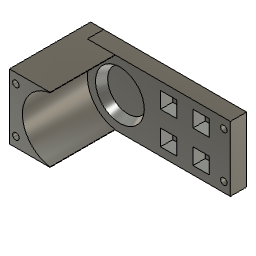
cementform_circle_80x40_plateA (Autodesk Fusion 360 design; units mm, degrees)
Autodesk Fusion 360 part; units mm, degrees
sketch "baseplate" plane through (0, 0, 0) normal (0, 1, 0) x (1, 0, 0)
  line L0 (0, 0) -> (80, 0)
  line L1 (80, 0) -> (80, -40)
  line L2 (80, -40) -> (0, -40)
  line L3 (0, -40) -> (0, 0)
  dimension "d1" = 40
  dimension "d2" = 80
  constraint horizontal L0
  constraint vertical L1
  constraint horizontal L2
  constraint vertical L3
  constraint coincident L0.start L3.end
  measures "d1" distance of L0.start L2.end
  measures "d2" distance of L0.start L0.end
extrude "Extrude1" add sketch "baseplate" along normal blind 10
sketch "outside_pryamid" plane through (0, 0, 0) normal (0, 1, 0) x (1, 0, 0)
  line L0 (45, -35) -> (55, -35)
  line L1 (55, -35) -> (55, -25)
  line L2 (55, -25) -> (45, -25)
  line L3 (45, -25) -> (45, -35)
  line L4 (65, -35) -> (75, -35)
  line L5 (75, -35) -> (75, -25)
  line L6 (75, -25) -> (65, -25)
  line L7 (65, -25) -> (65, -35)
  line L8 (45, -15) -> (55, -15)
  line L9 (55, -15) -> (55, -5)
  line L10 (55, -5) -> (45, -5)
  line L11 (45, -5) -> (45, -15)
  line L12 (65, -15) -> (75, -15)
  line L13 (75, -15) -> (75, -5)
  line L14 (75, -5) -> (65, -5)
  line L15 (65, -5) -> (65, -15)
  circle A0 centre (20, -20) radius 15
  dimension "d40" = 30
  constraint horizontal L0
  constraint vertical L1
  constraint horizontal L2
  constraint vertical L3
  constraint horizontal L4
  constraint vertical L5
  constraint horizontal L6
  constraint vertical L7
  constraint horizontal L8
  constraint vertical L9
  constraint horizontal L10
  constraint vertical L11
  constraint horizontal L12
  constraint vertical L13
  constraint horizontal L14
  constraint vertical L15
  measures "d40" diameter of A0
ref_plane "WorkPlane1" through (0, 5, 0) normal (0, 1, 0) x (0, 0, 1)
sketch "inside_pryamid" plane through (0, 5, 0) normal (0, 1, 0) x (1, 0, 0)
  line L0 (47.5, -7.5) -> (47.5, -10)
  line L1 (47.5, -12.5) -> (52.5, -12.5)
  line L2 (52.5, -7.5) -> (47.5, -7.5)
  line L3 (47.5, -10) -> (47.5, -12.5)
  line L4 (52.5, -12.5) -> (52.5, -7.5)
  line L5 (67.5, -10) -> (67.5, -12.5)
  line L6 (67.5, -12.5) -> (72.5, -12.5)
  line L7 (67.5, -7.5) -> (67.5, -10)
  line L8 (72.5, -12.5) -> (72.5, -7.5)
  line L9 (72.5, -7.5) -> (67.5, -7.5)
  line L10 (67.5, -10) -> (67.5, -12.5)
  line L11 (67.5, -12.5) -> (72.5, -12.5)
  line L12 (72.5, -12.5) -> (72.5, -7.5)
  line L13 (47.5, -7.5) -> (47.5, -10)
  line L14 (52.5, -12.5) -> (52.5, -7.5)
  line L15 (72.5, -7.5) -> (67.5, -7.5)
  line L16 (47.5, -10) -> (47.5, -12.5)
  line L17 (52.5, -7.5) -> (47.5, -7.5)
  line L18 (67.5, -7.5) -> (67.5, -10)
  line L19 (47.5, -12.5) -> (52.5, -12.5)
  line L20 (72.5, -32.5) -> (72.5, -27.5)
  line L21 (72.5, -27.5) -> (67.5, -27.5)
  line L22 (67.5, -30) -> (67.5, -32.5)
  line L23 (72.5, -27.5) -> (67.5, -27.5)
  line L24 (67.5, -27.5) -> (67.5, -30)
  line L25 (47.5, -30) -> (47.5, -32.5)
  line L26 (67.5, -27.5) -> (67.5, -30)
  line L27 (67.5, -30) -> (67.5, -32.5)
  line L28 (67.5, -32.5) -> (72.5, -32.5)
  line L29 (72.5, -32.5) -> (72.5, -27.5)
  line L30 (47.5, -32.5) -> (52.5, -32.5)
  line L31 (47.5, -32.5) -> (52.5, -32.5)
  line L32 (67.5, -32.5) -> (72.5, -32.5)
  line L33 (52.5, -32.5) -> (52.5, -27.5)
  line L34 (52.5, -27.5) -> (47.5, -27.5)
  line L35 (52.5, -27.5) -> (47.5, -27.5)
  line L36 (47.5, -30) -> (47.5, -32.5)
  line L37 (52.5, -32.5) -> (52.5, -27.5)
  line L38 (47.5, -27.5) -> (47.5, -30)
  line L39 (47.5, -27.5) -> (47.5, -30)
  circle A0 centre (20, -20) radius 12.5
  dimension "d42" = 25
  constraint perpendicular L1 L3
  constraint perpendicular L1 L4
  constraint perpendicular L2 L4
  constraint perpendicular L5 L6
  constraint perpendicular L6 L8
  constraint perpendicular L8 L9
  constraint perpendicular L16 L19
  constraint perpendicular L14 L19
  constraint perpendicular L14 L17
  constraint perpendicular L10 L11
  constraint perpendicular L11 L12
  constraint perpendicular L12 L15
  constraint perpendicular L25 L30
  constraint perpendicular L30 L37
  constraint perpendicular L35 L37
  constraint perpendicular L27 L32
  constraint perpendicular L29 L32
  constraint perpendicular L21 L29
  constraint perpendicular L31 L36
  constraint perpendicular L31 L33
  constraint perpendicular L33 L34
  constraint perpendicular L22 L28
  constraint perpendicular L20 L28
  constraint perpendicular L20 L23
  measures "d42" diameter of A0
loft "Loft9" cut profiles "inside_pryamid", "outside_pryamid" section 1 contours A0 section 2 contours A0
loft "Loft3" cut profiles "outside_pryamid", "inside_pryamid" section 1 contours L0 L1 L2 L3 section 2 contours L25 L30 L31 L33 L34 L35 L36 L37 L38 L39
loft "Loft4" cut profiles "inside_pryamid", "outside_pryamid" section 1 contours L20 L21 L22 L23 L24 L26 L27 L28 L29 L32 section 2 contours L4 L5 L6 L7
loft "Loft7" cut profiles "inside_pryamid", "outside_pryamid" section 1 contours L0 L1 L2 L3 L4 L13 L14 L16 L17 L19 section 2 contours L8 L9 L10 L11
loft "Loft8" cut profiles "inside_pryamid", "outside_pryamid" section 1 contours L5 L6 L7 L8 L9 L10 L11 L12 L15 L18 section 2 contours L12 L13 L14 L15
sketch "sidewall" plane through (0, 0, 0) normal (0, 1, 0) x (1, 0, 0)
  line L0 (-8, 0) -> (-8, -40)
  circle A0 centre (20, -20) radius 20
  line L1 (17, -20) -> (17, -40)
  line L2 (-8, -40) -> (17, -40)
  line L3 (17, -20) -> (17, 0)
  line L4 (-8, 0) -> (17, 0)
  dimension "d43" = 20
  dimension "d44" = 20
  constraint vertical L0
  measures "d43" distance of L1.start L1.end
  measures "d44" distance of L1.start L3.end
extrude "Extrude2" add sketch "sidewall" along normal blind -40 and the other way blind -10 contours L0 A0 L1 L2 L3 L4
sketch "sidemount" plane through (0, 0, 0) normal (0, 1, 0) x (1, 0, 0)
  line L0 (80, 0) -> (88, 0)
  line L1 (88, 0) -> (88, -40)
  line L2 (88, -40) -> (80, -40)
  line L3 (80, -40) -> (80, 0)
  constraint horizontal L0
  constraint vertical L1
  constraint horizontal L2
  constraint vertical L3
extrude "Extrude3" add sketch "sidemount" along normal blind 10
sketch "holes" plane through (0, 0, 0) normal (0, 1, 0) x (1, 0, 0)
  circle A0 centre (-4, -34) radius 2
  circle A1 centre (-4, -6) radius 2
  circle A2 centre (-4, -34) radius 3.4
  circle A3 centre (-4, -6) radius 3.4
  line L0 (88, 0) -> (84, 0)
  line L1 (84, 0) -> (84, -6)
  line L2 (84, -6) -> (88, -6)
  line L3 (88, -6) -> (88, 0)
  circle A4 centre (84, -34) radius 2
  circle A5 centre (84, -6) radius 2
  dimension "d19" = 4
  dimension "d20" = 4
  dimension "d21" = 6.8
  dimension "d22" = 6.8
  dimension "d25" = 4
  dimension "d26" = 6
  dimension "d27" = 4
  dimension "d28" = 4
  constraint concentric A0 A2
  constraint horizontal L0
  constraint vertical L1
  constraint horizontal L2
  constraint vertical L3
  constraint coincident L1.end L2.start
  measures "d19" diameter of A0
  measures "d20" diameter of A1
  measures "d21" diameter of A2
  measures "d22" diameter of A3
  measures "d25" distance of L0.start L0.end
  measures "d26" distance of L0.start L2.end
  measures "d27" diameter of A4
  measures "d28" diameter of A5
extrude "Extrude4" cut sketch "holes" against normal blind 50 contours A0 | A1
extrude "Extrude5" cut sketch "holes" along normal blind 40 contours L1 L2 A5 | L1 L2 A5 | A4
extrude "Extrude6" cut sketch "holes" along normal through all and the other way blind 44 contours A0 | A1
extrude "Extrude7" cut sketch "holes" along normal blind 10 and the other way blind -4 contours A2 | A3
